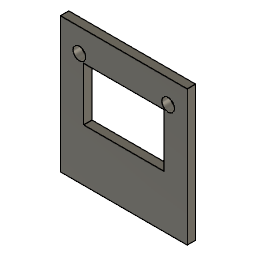
placa_baixo_ajuste_1 (Autodesk Fusion 360 design; units mm, degrees)
part number: 2025-10-18-19-38-59-563
Autodesk Fusion 360 part; units mm, degrees
note: some values were not read from the file. Set by a fixed rule: which sketch regions a step uses.
sketch "Sketch9" plane through (0, 0, 0) normal (0, 1, 0) x (1, 0, 0)
  line L0 (-5, 8) -> (25, 8)
  line L1 (25, 8) -> (25, -24)
  line L2 (25, -24) -> (-5, -24)
  line L3 (-5, -24) -> (-5, 8)
  line L4 (10, -18.5) -> (10, 8)
  line L5 (0.5, -4.382) -> (10, -4.382)
  line L6 (10, -4.382) -> (19.5, -4.382)
  line L7 (10, -18.5) -> (-0.5, -18.5)
  line L8 (10, -18.5) -> (20.5, -18.5)
  circle A0 centre (-0.5, -18.5) radius 1.5
  circle A1 centre (20.5, -18.5) radius 1.5
  line L9 (0.5, -4.382) -> (0.5, -17.382)
  line L10 (19.5, -4.382) -> (19.5, -17.382)
  line L11 (19.5, -17) -> (0.5, -17)
  dimension "d91" = 32
  dimension "d92" = 30
  dimension "d93" = 15
  dimension "d98" = 26.5
  dimension "d112" = 9.5
  dimension "d113" = 9.5
  dimension "d116" = 10.5
  dimension "d117" = 10.5
  dimension "d118" = 3
  dimension "d119" = 3
  dimension "d120" = 9.5
  dimension "d121" = 13
  constraint horizontal L0
  constraint vertical L1
  constraint horizontal L2
  constraint vertical L3
  constraint midpoint L0 L4.end
  constraint coincident L4 L5.end
  constraint perpendicular L4 L5
  constraint perpendicular L4 L6
  constraint perpendicular L4 L7
  constraint perpendicular L4 L8
  constraint coincident L7.end A0.centre
  constraint coincident L8.end A1.centre
  constraint coincident A0 L9.end
  constraint perpendicular L5 L9
  constraint perpendicular L6 L10
  constraint coincident L10 L11.start
  constraint coincident L9 L11.end
  constraint perpendicular L9 L11
  measures "d91" distance of L0.end L1.end
  measures "d92" distance of L0.start L0.end
  measures "d93" distance of L0.start L4.end
  measures "d98" distance of L4.end L4.start
  measures "d112" distance of L5.start L5.end
  measures "d113" distance of L5.end L6.end
  measures "d116" distance of L4.start L7.end
  measures "d117" distance of L4.start L8.end
  measures "d118" diameter of A0
  measures "d119" diameter of A1
  measures "d120" distance of L5.start L5.end
  measures "d121" distance of L5.start L9.end
extrude "Extrude13" add sketch "Sketch9" along normal blind 2 contours L0 L1 L2 L3 | L4 L7 A0 L9 L11 | L4 L8 A1 L10 L11
